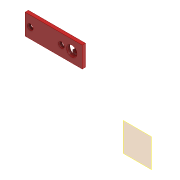
# Autodesk Inventor part: Odometry stop left
Saved by Autodesk Inventor 2020 (Build 240168000, 168)
## iProperties
Created: 2020-03-07
Part Number: Odometry stop left
Material: Generic
Document SubType Name: Modeling
Designer: ball
Density: 1 g/cm^3
Appearance: Default
Author: ball
Autodesk Inventor part; units mm, degrees
ref_plane "YZ Plane" through (0, 0, 0) normal (1, 0, 0) x (0, 1, 0)
ref_plane "XZ Plane" through (0, 0, 0) normal (0, 1, 0) x (-1, 0, 0)
ref_plane "XY Plane" through (0, 0, 0) normal (0, 0, 1) x (1, 0, 0)
ref_plane "Work Plane5" through (0, 0, 0) normal (0, 0, 1) x (1, 0, 0)
sketch "Sketch1" plane through (0, 0, 0) normal (0, 0, 1) x (1, 0, 0)
  arc A0 (-50, 35.3137) -> (-46, 35.3137) centre (-48, 35.3137) ccw construction
  arc A1 (-46, 40) -> (-50, 40) centre (-48, 40) ccw construction
  line L0 (-50, 35.3137) -> (-50, 40) construction
  line L1 (-46, 40) -> (-46, 35.3137) construction
  line L2 (-46.254, 38.8332) -> (-46.254, 35.3137)
  arc A2 (-49.746, 35.3137) -> (-46.254, 35.3137) centre (-48, 35.3137) ccw
  line L3 (-49.746, 35.3137) -> (-49.746, 38.8332)
  arc A3 (-49.746, 38.8332) -> (-46.254, 38.8332) centre (-48, 40) ccw
  point P0 (0, 0)
  dimension "d1" = 4.2
  constraints: 4 end point, 4 point on circle, 2 centre point, 1 coincident
  measures "d1" diameter of A3
extrude "Extrusion1" add sketch "Sketch1" against normal blind 2.5
ref_plane "Work Plane8" through (0, 0, 0) normal (0, 0, 1) x (1, 0, 0)
sketch "Sketch7" plane through (0, 0, 0) normal (0, 0, 1) x (1, 0, 0)
  line L0 (-40, 32) -> (-84, 32)
  line L1 (-84, 32) -> (-84, 48)
  line L2 (-84, 48) -> (-40, 48)
  line L3 (-40, 48) -> (-40, 32)
  circle A0 centre (-80, 40) radius 2.2
  arc A1 (-49.746, 38.8332) -> (-46.254, 38.8332) centre (-48, 40) ccw projected
  line L4 (-49.746, 35.3137) -> (-49.746, 38.8332) projected
  line L5 (-49.746, 36.4012) -> (-45.238, 36.4012) construction
  circle A2 centre (-56, 40) radius 2.2
  circle A3 centre (-48, 40) radius 4
  point P0 (0, 0)
  dimension "d34" = 16
  dimension "d35" = 4.4
  dimension "d37" = 32
  dimension "d39" = 8
  dimension "d41" = 36
  dimension "d42" = 8
  dimension "d49" = 4.4
  dimension "d50" = 8
  constraints: 10 end point, 3 centre point, 2 horizontal, 2 parallel, 1 coincident, 1 perpendicular, 1 point on line
  measures "d34" distance of L0.end L1.end
  measures "d35" diameter of A0
  measures "d37" distance of A0.centre A1.centre
  measures "d39" distance from line of L2 A0.centre
  measures "d41" distance from line of L1 A1.centre
  measures "d42" distance from line of L3 A1.centre
  measures "d49" diameter of A2
  measures "d50" diameter of A3
extrude "Extrusion7" add sketch "Sketch7" along normal blind 2.5
body "Solid1"
